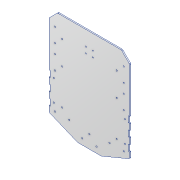
# Autodesk Inventor part: bottom
Saved by Autodesk Inventor 2020 (Build 240168000, 168)
## iProperties
Created: 2020-09-06
Part Number: bottom
Material: 알루미늄 6061
Document SubType Name: Sheet Metal
Designer: 이호석
Mass: 1857.26 g
Surface Area: 2848.33 cm^2
Volume: 687.874 cm^3
Density: 2.7 g/cm^3
Sheet Metal Rule: 기본값_mm
Appearance: 알루미늄 - 평지
Flat Pattern Width: 43 cm
Flat Pattern Length: 34 cm
Flat Pattern Area: 1462 cm^2
Sheet Metal Width: 430.000 mm
Sheet Metal Length: 340.000 mm
Sheet Metal Area: 146200.000 mm^2
Author: 이호석
Autodesk Inventor part; units mm, degrees
ref_plane "YZ Plane" through (0, 0, 0) normal (1, 0, 0) x (0, 1, 0)
ref_plane "XZ Plane" through (0, 0, 0) normal (0, 1, 0) x (-1, 0, 0)
ref_plane "XY Plane" through (0, 0, 0) normal (0, 0, 1) x (1, 0, 0)
sketch "스케치1" plane through (0, 0, 0) normal (0, 0, 1) x (1, 0, 0)
  line L0 (50, -215) -> (-50, -215)
  line L1 (-170, -165) -> (-170, 179.6447)
  line L2 (-134.6447, 215) -> (134.6447, 215)
  line L3 (170, 179.6447) -> (170, -165)
  line L4 (-170, -165) -> (-50, -215)
  line L5 (170, -165) -> (50, -215)
  line L6 (-134.6447, 215) -> (-170, 179.6447)
  line L7 (134.6447, 215) -> (170, 179.6447)
extrude "판1" add sketch "스케치1" along normal blind 5
sketch "스케치2" plane through (0, 0, 5) normal (0, 0, 1) x (1, 0, 0)
  line L0 (-134.6447, 215) -> (134.6447, 215) projected
  line L1 (0, 215) -> (0, 140)
  line L2 (19, 123.5) -> (-19, 123.5)
  line L3 (-19, 123.5) -> (-19, 156.5)
  line L4 (-19, 156.5) -> (19, 156.5)
  line L5 (19, 156.5) -> (19, 123.5)
  line L6 (19, 123.5) -> (-19, 156.5) construction
  line L7 (-19, 123.5) -> (19, 156.5) construction
  line L8 (14.5, 127.5) -> (-14.5, 127.5)
  line L9 (-14.5, 127.5) -> (-14.5, 152.5)
  line L10 (-14.5, 152.5) -> (14.5, 152.5)
  line L11 (14.5, 152.5) -> (14.5, 127.5)
  line L12 (14.5, 127.5) -> (-14.5, 152.5) construction
  line L13 (-14.5, 127.5) -> (14.5, 152.5) construction
  circle A0 centre (-14.5, 152.5) radius 2.1
  circle A1 centre (14.5, 152.5) radius 2.1
  circle A2 centre (-14.5, 127.5) radius 2.1
  circle A3 centre (14.5, 127.5) radius 2.1
  point P0 (0, 0)
  dimension "d11" = 75
  dimension "d215" = 38
  dimension "d216" = 33
  dimension "d217" = 29
  dimension "d218" = 25
  dimension "d219" = 4.2
  dimension "d220" = 4.2
  dimension "d221" = 4.2
  dimension "d222" = 4.2
  constraints: 26 end point, 5 midpoint, 4 centre point, 4 coincident, 4 parallel, 2 horizontal, 2 perpendicular, 1 vertical
  measures "d11" distance of L1.start L1.end
  measures "d215" distance of L3.end L4.end
  measures "d216" distance of L2.end L3.end
  measures "d217" distance of L9.end L10.end
  measures "d218" distance of L8.end L9.end
  measures "d219" diameter of A0
  measures "d220" diameter of A1
  measures "d221" diameter of A2
  measures "d222" diameter of A3
extrude "돌출1" cut sketch "스케치2" against normal through all contours A2 L9 L8 | L8 L9 A2 | A3 L11 L8 | L8 L11 A3 | A0 L10 L9 | L9 L10 A0 | A1 L10 L11 | L11 L10 A1
fillet "모서리 라운드1" radius 6 8 edges at (-134.6447, 215, 2.5) (134.6447, 215, 2.5) (170, 179.6447, 2.5) (170, -165, 2.5) (50, -215, 2.5) (-50, -215, 2.5) (-170, -165, 2.5) (-170, 179.6447, 2.5)
sketch "스케치3" plane through (0, 0, 5) normal (0, 0, 1) x (1, 0, 0)
  line L0 (48.8, -215) -> (-48.8, -215) projected
  line L1 (0, -215) -> (0, -205)
  line L2 (0, -205) -> (-15, -205)
  line L3 (-15, -205) -> (15, -205)
  line L4 (15, -205) -> (15, -175)
  line L5 (15, -175) -> (-15, -175)
  line L6 (-15, -175) -> (-15, -205)
  line L7 (130, -125) -> (130, 15)
  line L8 (-130, -125) -> (-130, 15)
  line L9 (-130, 15) -> (-160, 15)
  line L10 (-160, 15) -> (-160, 45)
  line L11 (-160, 45) -> (-130, 45)
  line L12 (-130, 45) -> (-130, 15)
  line L13 (130, 15) -> (160, 15)
  line L14 (160, 15) -> (160, 45)
  line L15 (160, 45) -> (130, 45)
  line L16 (130, 45) -> (130, 15)
  line L17 (130, 45) -> (130, 115)
  line L18 (-130, 45) -> (-130, 115)
  line L19 (-130, 115) -> (-160, 115)
  line L20 (-160, 115) -> (-160, 145)
  line L21 (-160, 145) -> (-130, 145)
  line L22 (-130, 145) -> (-130, 115)
  line L23 (130, 115) -> (160, 115)
  line L24 (160, 115) -> (160, 145)
  line L25 (160, 145) -> (130, 145)
  line L26 (130, 145) -> (130, 115)
  line L27 (165, -125) -> (170, -125)
  line L28 (170, -125) -> (170, -25)
  line L29 (170, -25) -> (165, -25)
  line L30 (165, -25) -> (165, -125)
  line L31 (-165, -125) -> (-170, -125)
  line L32 (-170, -125) -> (-170, -25)
  line L33 (-170, -25) -> (-165, -25)
  line L34 (-165, -25) -> (-165, -125)
  line L35 (-170, -125) -> (-170, -75)
  line L36 (-170, -161) -> (-170, 177.1594) projected
  line L37 (-170, -75) -> (170, -75)
  line L38 (0, -215) -> (0, -165)
  line L39 (0, -165) -> (-130, -165)
  line L40 (0, -165) -> (130, -165)
  line L41 (130, -165) -> (100, -165)
  line L42 (100, -165) -> (100, -135)
  line L43 (100, -135) -> (130, -135)
  line L44 (130, -135) -> (130, -165)
  line L45 (-130, -165) -> (-100, -165)
  line L46 (-100, -165) -> (-100, -135)
  line L47 (-100, -135) -> (-130, -135)
  line L48 (-130, -135) -> (-130, -165)
  line L49 (130, -135) -> (130, -125)
  line L50 (130, -125) -> (165, -125)
  line L51 (-130, -135) -> (-130, -125)
  line L52 (-130, -125) -> (-165, -125)
  line L53 (-100, -165) -> (-100, -162.5)
  line L54 (-100, -135) -> (-102.5, -135)
  line L55 (-130, -135) -> (-130, -137.5)
  line L56 (100, -165) -> (100, -162.5)
  line L57 (100, -135) -> (102.5, -135)
  line L58 (130, -135) -> (130, -137.5)
  line L59 (-15, -205) -> (-15, -202.5)
  line L60 (-15, -175) -> (-12.5, -175)
  line L61 (15, -175) -> (15, -177.5)
  line L62 (-130, -137.5) -> (-160, -137.5)
  line L63 (-160, -137.5) -> (-160, -162.5)
  line L64 (-160, -162.5) -> (-130, -162.5)
  line L65 (-130, -162.5) -> (-130, -137.5)
  line L66 (-102.5, -135) -> (-127.5, -135)
  line L67 (-127.5, -135) -> (-127.5, -105)
  line L68 (-127.5, -105) -> (-102.5, -105)
  line L69 (-102.5, -105) -> (-102.5, -135)
  line L70 (-100, -162.5) -> (-70, -162.5)
  line L71 (-70, -162.5) -> (-70, -137.5)
  line L72 (-70, -137.5) -> (-100, -137.5)
  line L73 (-100, -137.5) -> (-100, -162.5)
  line L74 (-12.5, -175) -> (12.5, -175)
  line L75 (12.5, -175) -> (12.5, -145)
  line L76 (12.5, -145) -> (-12.5, -145)
  line L77 (-12.5, -145) -> (-12.5, -175)
  line L78 (-15, -202.5) -> (-45, -202.5)
  line L79 (-45, -202.5) -> (-45, -177.5)
  line L80 (-45, -177.5) -> (-15, -177.5)
  line L81 (-15, -177.5) -> (-15, -202.5)
  line L82 (15, -177.5) -> (45, -177.5)
  line L83 (45, -177.5) -> (45, -202.5)
  line L84 (45, -202.5) -> (15, -202.5)
  line L85 (15, -202.5) -> (15, -177.5)
  line L86 (100, -162.5) -> (70, -162.5)
  line L87 (70, -162.5) -> (70, -137.5)
  line L88 (70, -137.5) -> (100, -137.5)
  line L89 (100, -137.5) -> (100, -162.5)
  line L90 (102.5, -135) -> (127.5, -135)
  line L91 (127.5, -135) -> (127.5, -105)
  line L92 (127.5, -105) -> (102.5, -105)
  line L93 (102.5, -105) -> (102.5, -135)
  line L94 (130, -137.5) -> (160, -137.5)
  line L95 (160, -137.5) -> (160, -162.5)
  line L96 (160, -162.5) -> (130, -162.5)
  line L97 (130, -162.5) -> (130, -137.5)
  line L98 (0, -175) -> (0, -160)
  line L99 (-15, -205) -> (-15, -190)
  line L100 (-15, -190) -> (-30, -190)
  line L101 (15, -190) -> (30, -190)
  line L102 (-100, -165) -> (-100, -150)
  line L103 (-100, -150) -> (-85, -150)
  line L104 (-130, -150) -> (-145, -150)
  line L105 (-115, -135) -> (-115, -120)
  line L106 (100, -165) -> (100, -150)
  line L107 (100, -150) -> (85, -150)
  line L108 (130, -165) -> (130, -150)
  line L109 (130, -150) -> (145, -150)
  line L110 (127.5, -135) -> (115, -135)
  line L111 (115, -135) -> (115, -120)
  circle A0 centre (-85, -150) radius 2.6
  circle A1 centre (-145, -150) radius 2.6
  circle A2 centre (-115, -120) radius 2.6
  circle A3 centre (-30, -190) radius 2.6
  circle A4 centre (30, -190) radius 2.6
  circle A5 centre (0, -160) radius 2.6
  circle A6 centre (85, -150) radius 2.6
  circle A7 centre (115, -120) radius 2.6
  circle A8 centre (145, -150) radius 2.6
  line L112 (-130, 15) -> (-145, 15)
  line L113 (-145, 15) -> (-145, 0)
  line L114 (130, 15) -> (145, 15)
  line L115 (145, 15) -> (145, 0)
  line L116 (-145, 45) -> (-145, 60)
  line L117 (-145, 115) -> (-145, 100)
  line L118 (-145, 145) -> (-145, 160)
  line L119 (145, 45) -> (145, 60)
  line L120 (145, 115) -> (145, 100)
  line L121 (145, 145) -> (145, 160)
  line L122 (130, 145) -> (130, 130)
  line L123 (130, 130) -> (115, 130)
  line L124 (-130, 130) -> (-115, 130)
  line L125 (-130, 30) -> (-115, 30)
  line L126 (130, 30) -> (115, 30)
  circle A9 centre (145, 0) radius 2.6
  circle A10 centre (115, 30) radius 2.6
  circle A11 centre (145, 60) radius 2.6
  circle A12 centre (145, 100) radius 2.6
  circle A13 centre (115, 130) radius 2.6
  circle A14 centre (145, 160) radius 2.6
  circle A15 centre (-145, 100) radius 2.6
  circle A16 centre (-115, 130) radius 2.6
  circle A17 centre (-145, 160) radius 2.6
  circle A18 centre (-145, 60) radius 2.6
  circle A19 centre (-115, 30) radius 2.6
  circle A20 centre (-145, 0) radius 2.6
  point P0 (0, 0)
  dimension "d63" = 2.5
  dimension "d64" = 2.5
  dimension "d65" = 2.5
  dimension "d66" = 2.5
  dimension "d67" = 2.5
  dimension "d68" = 2.5
  dimension "d69" = 2.5
  dimension "d70" = 2.5
  dimension "d71" = 2.5
  dimension "d72" = 30
  dimension "d73" = 25
  dimension "d74" = 25
  dimension "d75" = 30
  dimension "d76" = 30
  dimension "d77" = 25
  dimension "d78" = 25
  dimension "d79" = 30
  dimension "d80" = 30
  dimension "d81" = 25
  dimension "d82" = 30
  dimension "d83" = 25
  dimension "d84" = 30
  dimension "d85" = 25
  dimension "d86" = 25
  dimension "d87" = 30
  dimension "d88" = 30
  dimension "d89" = 25
  dimension "d90" = 15
  dimension "d91" = 15
  dimension "d92" = 15
  dimension "d93" = 15
  dimension "d94" = 15
  dimension "d97" = 15
  dimension "d98" = 15
  dimension "d99" = 5.2
  dimension "d100" = 5.2
  dimension "d101" = 5.2
  dimension "d102" = 5.2
  dimension "d103" = 5.2
  dimension "d104" = 5.2
  dimension "d105" = 5.2
  dimension "d106" = 5.2
  dimension "d107" = 15
  dimension "d108" = 15
  dimension "d109" = 15
  dimension "d110" = 15
  dimension "d111" = 15
  dimension "d112" = 15
  dimension "d113" = 15
  dimension "d114" = 15
  dimension "d115" = 15
  dimension "d116" = 15
  dimension "d117" = 15
  dimension "d118" = 15
  dimension "d119" = 15
  dimension "d120" = 5.2
  dimension "d121" = 5.2
  dimension "d122" = 5.2
  dimension "d123" = 5.2
  dimension "d124" = 5.2
  constraints: 250 end point, 36 parallel, 30 perpendicular, 24 horizontal, 23 midpoint, 21 centre point, 21 coincident, 15 vertical, 11 point on line
  measures "d63" distance of L45.end L53.end
  measures "d64" distance of L46.end L54.end
  measures "d65" distance of L47.end L55.end
  measures "d66" distance of L41.end L56.end
  measures "d67" distance of L42.end L57.end
  measures "d68" distance of L43.end L58.end
  measures "d69" distance of L2.end L59.end
  measures "d70" distance of L5.end L60.end
  measures "d71" distance of L4.end L61.end
  measures "d72" distance of L64.end L63.end
  measures "d73" distance of L63.end L62.end
  measures "d74" distance of L67.end L68.end
  measures "d75" distance of L66.end L67.end
  measures "d76" distance of L72.end L71.end
  measures "d77" distance of L71.end L70.end
  measures "d78" distance of L76.end L75.end
  measures "d79" distance of L75.end L74.end
  measures "d80" distance of L79.end L80.end
  measures "d81" distance of L78.end L79.end
  measures "d82" distance of L83.end L84.end
  measures "d83" distance of L82.end L83.end
  measures "d84" distance of L87.end L88.end
  measures "d85" distance of L86.end L87.end
  measures "d86" distance of L92.end L91.end
  measures "d87" distance of L91.end L90.end
  measures "d88" distance of L95.end L96.end
  measures "d89" distance of L94.end L95.end
  measures "d90" distance of L98.start L98.end
  measures "d91" distance of L2.end L99.end
  measures "d92" distance of L99.end L100.end
  measures "d93" distance of L101.start L101.end
  measures "d94" distance of L105.start L105.end
  measures "d97" distance of L41.end L106.end
  measures "d98" distance of L106.end L107.end
  measures "d99" diameter of A0
  measures "d100" diameter of A2
  measures "d101" diameter of A3
  measures "d102" diameter of A4
  measures "d103" diameter of A5
  measures "d104" diameter of A6
  measures "d105" diameter of A7
  measures "d106" diameter of A8
  measures "d107" distance of L8.end L112.end
  measures "d108" distance of L112.end L113.end
  measures "d109" distance of L7.end L114.end
  measures "d110" distance of L116.start L116.end
  measures "d111" distance of L117.start L117.end
  measures "d112" distance of L118.start L118.end
  measures "d113" distance of L119.start L119.end
  measures "d114" distance of L120.start L120.end
  measures "d115" distance of L121.start L121.end
  measures "d116" distance of L25.end L122.end
  measures "d117" distance of L122.end L123.end
  measures "d118" distance of L124.start L124.end
  measures "d119" distance of L126.start L126.end
  measures "d120" diameter of A9
  measures "d121" diameter of A10
  measures "d122" diameter of A11
  measures "d123" diameter of A12
  measures "d124" diameter of A14
extrude "돌출2" cut sketch "스케치3" against normal through all contours A0 | A1 | A2 | A3 | A4 | A5 | A6 | A7 | A8 | A9 | A10 | A11 | A12 | A13 | A14 | A15 | A16 | A17 | A18 | A19 | A20
sketch "스케치5" plane through (0, 0, 5) normal (0, 0, 1) x (1, 0, 0)
  line L0 (48.8, -215) -> (-48.8, -215) projected
  line L1 (0, -215) -> (0, -140)
  line L2 (0, -140) -> (-165, -140)
  line L3 (0, -140) -> (165, -140)
  line L4 (-165, -140) -> (-170, -140)
  line L5 (-170, -140) -> (-170, -10)
  line L6 (-170, -10) -> (-165, -10)
  line L7 (-165, -10) -> (-165, -140)
  line L8 (165, -140) -> (170, -140)
  line L9 (170, -140) -> (170, -10)
  line L10 (170, -10) -> (165, -10)
  line L11 (165, -10) -> (165, -140)
  line L12 (165, -140) -> (165, -135)
  line L13 (165, -10) -> (165, -15)
  line L14 (-165, -10) -> (-165, -15)
  line L15 (-165, -140) -> (-165, -135)
  line L16 (-165, -15) -> (-135, -15)
  line L17 (-135, -15) -> (-135, -45)
  line L18 (-135, -45) -> (-165, -45)
  line L19 (-165, -45) -> (-165, -15)
  line L20 (-165, -135) -> (-135, -135)
  line L21 (-135, -135) -> (-135, -105)
  line L22 (-135, -105) -> (-165, -105)
  line L23 (-165, -105) -> (-165, -135)
  line L24 (165, -135) -> (135, -135)
  line L25 (135, -135) -> (135, -105)
  line L26 (135, -105) -> (165, -105)
  line L27 (165, -105) -> (165, -135)
  line L28 (165, -15) -> (135, -15)
  line L29 (135, -15) -> (135, -45)
  line L30 (135, -45) -> (165, -45)
  line L31 (165, -45) -> (165, -15)
  line L32 (165, -15) -> (165, -30)
  line L33 (165, -30) -> (150, -30)
  line L34 (165, -120) -> (150, -120)
  line L35 (-165, -120) -> (-150, -120)
  line L36 (-165, -30) -> (-150, -30)
  circle A0 centre (-150, -30) radius 2.6
  circle A1 centre (-150, -120) radius 2.6
  circle A2 centre (150, -120) radius 2.6
  circle A3 centre (150, -30) radius 2.6
  line L37 (-170, -140) -> (-170, -114)
  line L38 (-170, -161) -> (-170, 177.1594) projected
  line L39 (-170, -114) -> (-170, -88)
  line L40 (-170, -88) -> (-170, -62)
  line L41 (-170, -62) -> (-170, -36)
  line L42 (-170, -36) -> (-170, -10)
  line L43 (-170, -36) -> (-165, -36)
  line L44 (-170, -62) -> (-165, -62)
  line L45 (-170, -88) -> (-165, -88)
  line L46 (-170, -114) -> (-165, -114)
  line L47 (170, -140) -> (170, -114)
  line L48 (170, 177.1594) -> (170, -161) projected
  line L49 (170, -114) -> (170, -88)
  line L50 (170, -88) -> (170, -62)
  line L51 (170, -62) -> (170, -36)
  line L52 (170, -36) -> (170, -10)
  line L53 (170, -36) -> (165, -36)
  line L54 (170, -62) -> (165, -62)
  line L55 (170, -88) -> (165, -88)
  line L56 (170, -114) -> (165, -114)
  point P0 (0, 0)
  dimension "d192" = 5
  dimension "d193" = 130
  dimension "d194" = 5
  dimension "d195" = 130
  dimension "d196" = 5
  dimension "d197" = 5
  dimension "d198" = 5
  dimension "d199" = 5
  dimension "d200" = 30
  dimension "d201" = 30
  dimension "d202" = 30
  dimension "d203" = 30
  dimension "d204" = 30
  dimension "d205" = 30
  dimension "d206" = 30
  dimension "d207" = 30
  dimension "d208" = 15
  dimension "d209" = 5.2
  dimension "d210" = 5.2
  dimension "d211" = 5.2
  dimension "d212" = 5.2
  dimension "d223" = 26
  dimension "d224" = 26
  dimension "d225" = 26
  dimension "d226" = 26
  dimension "d227" = 26
  dimension "d228" = 5
  dimension "d229" = 26
  dimension "d230" = 26
  dimension "d231" = 26
  dimension "d232" = 26
  dimension "d233" = 26
  constraints: 108 end point, 20 point on line, 16 perpendicular, 14 equal length, 9 horizontal, 5 midpoint, 4 centre point, 4 coincident, 1 vertical
  measures "d192" distance of L5.end L6.end
  measures "d193" distance of L4.end L5.end
  measures "d194" distance of L10.end L9.end
  measures "d195" distance of L9.end L8.end
  measures "d196" distance of L3.end L12.end
  measures "d197" distance of L10.end L13.end
  measures "d198" distance of L6.end L14.end
  measures "d199" distance of L2.end L15.end
  measures "d200" distance of L17.end L18.end
  measures "d201" distance of L16.end L17.end
  measures "d202" distance of L22.end L21.end
  measures "d203" distance of L21.end L20.end
  measures "d204" distance of L25.end L26.end
  measures "d205" distance of L24.end L25.end
  measures "d206" distance of L30.end L29.end
  measures "d207" distance of L29.end L28.end
  measures "d208" distance of L13.end L32.end
  measures "d209" diameter of A0
  measures "d210" diameter of A1
  measures "d211" diameter of A2
  measures "d212" diameter of A3
  measures "d223" distance of L4.end L37.end
  measures "d224" distance of L37.end L39.end
  measures "d225" distance of L39.end L40.end
  measures "d226" distance of L40.end L41.end
  measures "d227" distance of L41.end L5.end
  measures "d228" distance of L41.end L43.end
  measures "d229" distance of L8.end L47.end
  measures "d230" distance of L47.end L49.end
  measures "d231" distance of L49.end L50.end
  measures "d232" distance of L50.end L51.end
  measures "d233" distance of L51.end L9.end
extrude "돌출3" cut sketch "스케치5" against normal through all contours L4 L5 L46 L7 | L5 L44 L7 L45 | L5 L6 L7 L43 | L11 L56 L9 L8 | L55 L11 L54 L9 | L53 L11 L10 L9 | A0 | A1 | A2 | A3
equation "\"TransitionRadius\" = BendRadius"
equation "\"BendRadius\" = 5"
